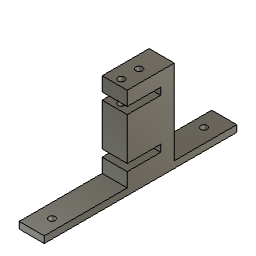
FixedArmHolder v1 (Autodesk Fusion 360 design; units mm, degrees)
Autodesk Fusion 360 part; units mm, degrees
sketch "Sketch1" plane through (0, 0, 0) normal (0, 0, 1) x (1, 0, 0)
  line L0 (30.2, 81.2805) -> (41.5, 81.2805)
  line L1 (41.5, 81.2805) -> (41.5, -5.4195)
  line L2 (41.5, -5.4195) -> (30.2, -5.4195)
  line L3 (30.2, -5.4195) -> (30.2, 81.2805)
  circle A0 centre (36.5, 3.0805) radius 1.5
  circle A1 centre (35.2, 72.7805) radius 1.5
  dimension "d1" = 1.3
  dimension "d2" = 69.7
  dimension "d3" = 3
  dimension "d4" = 3
  dimension "d5" = 5
  dimension "d6" = 5
  dimension "d7" = 8.5
  dimension "d8" = 8.5
  constraint horizontal L0
  constraint vertical L1
  constraint horizontal L2
  constraint vertical L3
  measures "d1" horizontal distance of A0.centre A1.centre
  measures "d2" vertical distance of A0.centre A1.centre
  measures "d3" diameter of A1
  measures "d4" diameter of A0
  measures "d5" distance of L1 A0.centre
  measures "d6" distance of L3 A1.centre
  measures "d7" distance of L0 A1.centre
  measures "d8" distance of L2 A0.centre
extrude "Extrude1" add sketch "Sketch1" along normal blind 3
sketch "Sketch2" plane through (0, 0, 3) normal (0, 0, 1) x (-1, 0, 0)
  circle A0 centre (-36.5, -3.0805) radius 1.5
  circle A1 centre (-35.2, -72.7805) radius 1.5
  line L0 (-30.2, 5.4195) -> (-41.5, 5.4195)
  line L1 (-41.5, 5.4195) -> (-41.5, -81.2805)
  line L2 (-41.5, -81.2805) -> (-30.2, -81.2805)
  line L3 (-30.2, -81.2805) -> (-30.2, 5.4195)
  line L4 (-30.2, -53.1183) -> (-41.5, -53.1183)
  line L5 (-41.5, -53.1183) -> (-41.5, -31.956)
  line L6 (-41.5, -31.956) -> (-30.2, -31.956)
  line L7 (-30.2, -31.956) -> (-30.2, -53.1183)
  constraint horizontal L4
  constraint vertical L5
  constraint horizontal L6
  constraint vertical L7
  constraint coincident L1 L5.end
  constraint coincident L3 L4.start
extrude "Extrude2" add sketch "Sketch2" along normal blind 38.1 contours L1 L3 L4 L5 L6 L7
sketch "Sketch3" plane through (41.5, 0, 0) normal (1, 0, 0) x (0, 1, 0)
  line L0 (-5.4195, 0) -> (81.2805, 0)
  line L1 (81.2805, 0) -> (81.2805, 3)
  line L2 (81.2805, 3) -> (53.1183, 3)
  line L3 (53.1183, 3) -> (53.1183, 41.1)
  line L4 (53.1183, 41.1) -> (31.956, 41.1)
  line L5 (31.956, 41.1) -> (31.956, 3)
  line L6 (31.956, 3) -> (-5.4195, 3)
  line L7 (-5.4195, 3) -> (-5.4195, 0)
  line L8 (31.956, 34.75) -> (47, 34.75)
  line L9 (47, 34.75) -> (47, 31.575)
  line L10 (47, 31.575) -> (31.956, 31.575)
  line L11 (31.956, 31.575) -> (31.956, 34.75)
  line L12 (31.956, 12.525) -> (47, 12.525)
  line L13 (47, 12.525) -> (47, 9.35)
  line L14 (47, 9.35) -> (31.956, 9.35)
  line L15 (31.956, 9.35) -> (31.956, 12.525)
  dimension "d13" = 3.175
  dimension "d14" = 3.175
  dimension "d15" = 19.05
  dimension "d16" = 6.35
  constraint horizontal L8
  constraint vertical L9
  constraint horizontal L10
  constraint vertical L11
  constraint coincident L5 L8.start
  constraint horizontal L12
  constraint vertical L13
  constraint horizontal L14
  constraint vertical L15
  constraint coincident L5 L12.start
  measures "d13" distance of L8 L10
  measures "d14" distance of L12.start L14.end
  measures "d15" distance of L10 L12
  measures "d16" distance of L4 L8
extrude "Extrude3" cut sketch "Sketch3" against normal blind 15 contours L5 L12 L13 L14 L15 | L5 L8 L9 L10 L11
sketch "Sketch4" plane through (0, 0, 41.1) normal (0, 0, 1) x (-1, 0, 0)
  line L0 (-30.2, -31.956) -> (-41.5, -31.956)
  line L1 (-41.5, -31.956) -> (-41.5, -53.1183)
  line L2 (-41.5, -53.1183) -> (-30.2, -53.1183)
  line L3 (-30.2, -53.1183) -> (-30.2, -31.956)
  circle A0 centre (-35.85, -34.956) radius 1.5
  circle A1 centre (-35.85, -42.956) radius 1.5
  dimension "d19" = 3
  dimension "d20" = 3
  dimension "d21" = 3
  dimension "d22" = 8
  measures "d19" diameter of A0
  measures "d20" diameter of A1
  measures "d21" distance of L0 A0.centre
  measures "d22" distance of A0.centre A1.centre
extrude "Extrude4" cut sketch "Sketch4" against normal blind 30 contours A0 | A1
